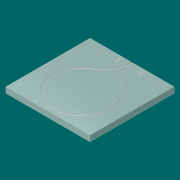
# Autodesk Inventor part: Scintillator Tile
Saved by Autodesk Inventor 2016 (Build 200138000, 138)
## iProperties
Created: 2015-08-14
Part Number: Scintillator Tile
Material: ABS Plastic
Document SubType Name: Modeling
Designer: Cosmic
Density: 1.06 g/cm^3
Appearance: Clear
Author: Cosmic
Autodesk Inventor part; units mm, degrees
ref_plane "YZ Plane" through (0, 0, 0) normal (1, 0, 0) x (0, 1, 0)
ref_plane "XZ Plane" through (0, 0, 0) normal (0, 1, 0) x (-1, 0, 0)
ref_plane "XY Plane" through (0, 0, 0) normal (0, 0, 1) x (1, 0, 0)
sketch "Sketch1" plane through (0, 0, 0) normal (0, 0, 1) x (1, 0, 0)
  line L0 (-72.5, -72.5) -> (72.5, -72.5)
  line L1 (72.5, -72.5) -> (72.5, 72.5)
  line L2 (72.5, 72.5) -> (-72.5, 72.5)
  line L3 (-72.5, 72.5) -> (-72.5, -72.5)
  line L4 (-72.5, -72.5) -> (72.5, 72.5) construction
  line L5 (72.5, -72.5) -> (-72.5, 72.5) construction
  point P0 (0, 0)
  dimension "d0" = 145
  dimension "d1" = 145
  constraints: 12 end point, 2 midpoint, 2 parallel, 1 horizontal, 1 perpendicular
  measures "d0" distance of L2.end L1.end
  measures "d1" distance of L1.end L0.end
extrude "Extrusion1" add sketch "Sketch1" along normal blind 10
sketch "Sketch6" plane through (0, 0, 10) normal (0, 0, 1) x (1, 0, 0)
  line L0 (-72.5, -72.5) -> (72.5, -72.5) projected
  line L1 (72.5, -72.5) -> (72.5, 72.5) projected
  line L2 (72.5, 72.5) -> (-72.5, 72.5) projected
  line L3 (-72.5, 72.5) -> (-72.5, -72.5) projected
  arc A0 (-23.9233, 28.9664) -> (23.9233, 28.9664) centre (0, -14.3686) ccw
  arc A1 (-24.5516, 30.1045) -> (-31.1763, 25.7397) centre (0, -14.3686) ccw
  arc A2 (-24.5516, 30.1045) -> (-1.3, 69.5) centre (-46.3, 69.5) ccw
  arc A3 (24.5516, 30.1045) -> (72.5, 32.9137) centre (46.3, 69.5) ccw
  arc A4 (-31.1763, 25.7397) -> (-23.9233, 28.9664) centre (-46.3, 69.5) ccw
  arc A5 (17.3281, 33.3846) -> (23.9233, 28.9664) centre (46.3, 69.5) ccw
  line L4 (-46.3, 69.5) -> (46.3, 69.5)
  arc A6 (-72.5, 32.9137) -> (-24.5516, 30.1045) centre (-46.3, 69.5) ccw
  arc A7 (-72.5, 31.3261) -> (-31.1763, 25.7397) centre (-46.3, 69.5) ccw
  arc A8 (-1.3, 69.5) -> (-72.5, 32.9137) centre (-46.3, 69.5) ccw
  arc A9 (-23.9233, 28.9664) -> (-17.3281, 33.3846) centre (-46.3, 69.5) ccw
  arc A10 (23.9233, 28.9664) -> (-23.9233, 28.9664) centre (0, -14.3686) ccw
  arc A11 (-17.3281, 33.3846) -> (-24.5516, 30.1045) centre (0, -14.3686) ccw
  arc A12 (-31.1763, 25.7397) -> (31.1763, 25.7397) centre (0, -14.3686) ccw
  arc A13 (17.3281, 33.3846) -> (-17.3281, 33.3846) centre (0, -14.3686) ccw
  arc A14 (24.5516, 30.1045) -> (17.3281, 33.3846) centre (0, -14.3686) ccw
  arc A15 (0, 69.5) -> (17.3281, 33.3846) centre (46.3, 69.5) ccw
  arc A16 (1.3, 69.5) -> (24.5516, 30.1045) centre (46.3, 69.5) ccw
  arc A17 (0, 69.5) -> (-72.5, 31.3261) centre (-46.3, 69.5) ccw
  arc A18 (-17.3281, 33.3846) -> (0, 69.5) centre (-46.3, 69.5) ccw
  arc A19 (23.9233, 28.9664) -> (31.1763, 25.7397) centre (46.3, 69.5) ccw
  arc A20 (31.1763, 25.7397) -> (24.5516, 30.1045) centre (0, -14.3686) ccw
  arc A21 (31.1763, 25.7397) -> (72.5, 31.3261) centre (46.3, 69.5) ccw
  arc A22 (72.5, 32.9137) -> (1.3, 69.5) centre (46.3, 69.5) ccw
  arc A23 (72.5, 31.3261) -> (0, 69.5) centre (46.3, 69.5) ccw
  point P0 (0, 0)
  point P1 (0, 69.5)
  dimension "d44" = 1.3
  dimension "d45" = 1.3
  dimension "d46" = 1.3
  dimension "d47" = 90
  dimension "d48" = 90
  dimension "d49" = 99
  dimension "d50" = 3
  dimension "d51" = 72.5
  constraints: 49 point on circle, 24 centre point, 6 point on line, 3 tangent, 2 end point, 1 horizontal, 1 midpoint
  measures "d44" radial gap between concentric circles of A4 A2
  measures "d45" radial gap between concentric circles of A3 A5
  measures "d46" radial gap between concentric circles of A0 A1
  measures "d47" diameter of A2
  measures "d48" diameter of A3
  measures "d49" diameter of A0
  measures "d50" distance between parallel lines of L2 L4
  measures "d51" distance from line of L3 point (0, 69.5)
extrude "Extrusion8" cut sketch "Sketch6" against normal blind 1.3 contours A17 L2 A8 L3 | L1 A22 L2 A23 | A1 A11 A9 A4 | A4 A0 A19 A12 | A17 L4 A8 L2 | A19 A5 A14 A20 | L2 A22 L4 A23 | A2 L4 A18 A11 | L4 A16 A14 A15
sketch "Sketch7" plane through (0, 0, 10) normal (0, 0, 1) x (1, 0, 0)
  line L0 (-72.5, -72.5) -> (72.5, -72.5) projected
  line L1 (-72.5, 72.5) -> (-72.5, -72.5) projected
  line L2 (72.5, 72.5) -> (-72.5, 72.5) projected
  line L3 (72.5, -72.5) -> (72.5, 72.5) projected
  line L4 (-5, 72.5) -> (5, 72.5)
  line L5 (5, 72.5) -> (5, 69.5)
  line L6 (5, 69.5) -> (-5, 69.5)
  line L7 (-5, 69.5) -> (-5, 72.5)
  point P0 (0, 0)
  dimension "d54" = 10
  dimension "d55" = 67.5
  dimension "d56" = 3
  constraints: 8 end point, 2 parallel, 1 horizontal, 1 perpendicular, 1 point on line
  measures "d54" distance between parallel lines of L5 L7
  measures "d55" distance between parallel lines of L3 L5
  measures "d56" distance between parallel lines of L2 L6
extrude "Extrusion9" add sketch "Sketch7" against normal up to surface (10 mm away) contours L2 L5 L6 L7
sketch "Sketch8" plane through (0, 0, 10) normal (0, 0, 1) x (1, 0, 0)
  line L0 (72.5, 72.5) -> (-72.5, 72.5) projected
  line L1 (72.5, -72.5) -> (72.5, 72.5) projected
  line L2 (-72.5, -72.5) -> (72.5, -72.5) projected
  line L3 (-72.5, 72.5) -> (-72.5, -72.5) projected
  line L4 (-1.3, 72.5) -> (1.3, 72.5)
  line L5 (1.3, 72.5) -> (1.3, 62.5)
  line L6 (1.3, 62.5) -> (-1.3, 62.5)
  line L7 (-1.3, 62.5) -> (-1.3, 72.5)
  point P0 (0, 0)
  dimension "d59" = 2.6
  dimension "d60" = 10
  dimension "d61" = 71.2
  constraints: 8 end point, 2 parallel, 1 horizontal, 1 perpendicular, 1 point on line
  measures "d59" distance between parallel lines of L5 L7
  measures "d60" distance between parallel lines of L0 L6
  measures "d61" distance between parallel lines of L3 L7
extrude "Extrusion10" cut sketch "Sketch8" against normal up to surface (1.3 mm away) contours L5 L6 L7 L0
sketch "Sketch9" plane through (-72.5, 72.5, 0) normal (0, 1, 0) x (1, 0, 0)
  line L0 (71.2, -8.7) -> (73.8, -8.7) projected
  line L1 (145, -10) -> (73.8, -10) projected
  line L2 (145, 0) -> (145, -10) projected
  line L3 (145, 0) -> (0, 0) projected
  line L4 (0, 0) -> (0, -10) projected
  line L5 (96.4233, -10) -> (73.0322, -10) projected
  line L6 (75.525, -10) -> (69.475, -10)
  line L7 (69.475, -10) -> (69.475, -5.67)
  line L8 (69.475, -5.67) -> (75.525, -5.67)
  line L9 (75.525, -5.67) -> (75.525, -10)
  line L10 (72.5, -5.67) -> (72.5, -10)
  line L11 (73.0322, -10) -> (71.9678, -10) projected
  line L12 (71.2, -10) -> (71.2, -8.7) projected
  line L13 (73.8, -8.7) -> (73.8, -10) projected
  line L14 (71.2, -10) -> (0, -10) projected
  point P0 (72.5, 0)
  point P1 (76.3, -7)
  dimension "d64" = 4.33
  dimension "d65" = 6.05
  dimension "d66" = 72.5
  constraints: 10 end point, 2 midpoint, 2 parallel, 2 perpendicular, 1 horizontal, 2 other
  measures "d64" distance of L8.end L6.start
  measures "d65" distance of L7.end L8.end
  measures "d66" distance between parallel lines of L4 L10
extrude "Extrusion11" [suppressed]
fillet "Fillet1" radius 0.65 7 edges at (-1.3, 71, 8.7) (-27.9492, 28.0516, 8.7) (7.5464, 46.6273, 8.7) (1.3, 71, 8.7) (0, -63.8686, 8.7) (-8.3257, 43.0114, 8.7) (8.3257, 43.0114, 8.7)
sketch "Sketch10" plane through (-72.5, 72.5, 0) normal (0, 1, 0) x (1, 0, 0)
  line L0 (92.5, -6) -> (52.5, -6)
  line L1 (71.2, -10) -> (0, -10) projected
  line L2 (0, -10) -> (145, -10) projected
  line L3 (145, -10) -> (73.8, -10) projected
  line L4 (73.8, -10) -> (97.0516, -10) projected
  line L5 (97.0516, -10) -> (47.9484, -10) projected
  line L6 (47.9484, -10) -> (71.2, -10) projected
  point P0 (72.5, 0)
  dimension "d70" = 4
  dimension "d71" = 20
  dimension "d72" = 20
  constraints: 2 end point, 1 horizontal
  measures "d70" distance from line of L1 L0.end
  measures "d71" horizontal distance of L0.end point (72.5, 0)
  measures "d72" horizontal distance of point (72.5, 0) L0.start
hole "Hole1" at (20, 72.5, 6) at (-20, 72.5, 6) direction (0, -1, 0) diameter 2.459 depth 8.8 tip angle 118 thread size "M3x0.5" class "6H" standard "ISO Metric profile"
equation "\"d0\" = ScintillatorWidth"
equation "\"d1\" = ScintillatorHeight"
equation "\"d2\" = ScintillatorThickness"
equation "\"d44\" = OpticalFiberDiameter + 2 * OpticalFiberClearence"
equation "\"d45\" = OpticalFiberDiameter + 2 * OpticalFiberClearence"
equation "\"d46\" = OpticalFiberDiameter + 2 * OpticalFiberClearence"
equation "\"d47\" = LoopSmallTrackDiameter"
equation "\"d48\" = LoopSmallTrackDiameter"
equation "\"d50\" = ScintillatorEdgeClearence"
equation "\"d51\" = 0.5 * ScintillatorWidth"
equation "\"d52\" = ShallowTrackDepth"
equation "\"MPPCDepth\" = 0"
equation "\"MPPCWidth\" = 5.9"
equation "\"MPPCHeight\" = 6.55"
equation "\"MPPCClearence\" = 0.075"
equation "\"LongFiberAngle\" = 30deg"
equation "\"LargeTrackRatio\" = 3"
equation "\"ShortFiberAngle\" = 78deg"
equation "\"FiberEdgeOffsett\" = 5"
equation "\"MPPCSensorOffsett\" = 2.105"
equation "\"ScintillatorWidth\" = 145"
equation "\"ShallowTrackDepth\" = 1.3"
equation "\"MountingScrewDepth\" = 4"
equation "\"ScintillatorHeight\" = 145"
equation "\"SmallTrackDiameter\" = 175"
equation "\"FiberSensorClerence\" = 0.5"
equation "\"LoopLargeTrackRatio\" = 1.1"
equation "\"MPPCSensorClearence\" = 1.45"
equation "\"MountingScrewOffsett\" = 20"
equation "\"OpticalFiberDiameter\" = 1"
equation "\"OpticalFiberClearence\" = 0.15"
equation "\"ScintillatorThickness\" = 10"
equation "\"LoopSmallTrackDiameter\" = 90"
equation "\"ScintillatorEdgeClearence\" = 3"
equation "\"d55\" = 0.5 * ScintillatorWidth - 0.5 * d54"
equation "\"d56\" = ScintillatorEdgeClearence"
equation "\"d57\" = ShallowTrackDepth"
equation "\"d59\" = 4 * OpticalFiberClearence + 2 * OpticalFiberDiameter"
equation "\"d61\" = 0.5 * ScintillatorWidth - 2 * OpticalFiberClearence - OpticalFiberDiameter"
equation "\"d62\" = ShallowTrackDepth"
equation "\"d65\" = MPPCWidth + 2 * MPPCClearence"
equation "\"d66\" = 0.5 * ScintillatorWidth"
equation "\"d69\" = OpticalFiberClearence + 0.5 * OpticalFiberDiameter"
equation "\"d70\" = MountingScrewDepth"
equation "\"d71\" = MountingScrewOffsett"
equation "\"d72\" = MountingScrewOffsett"
equation "\"d5\" = OpticalFiberDiameter + 2 * OpticalFiberClearence"
equation "\"d21\" = d5"
equation "\"d22\" = d5"
body "Solid1"
